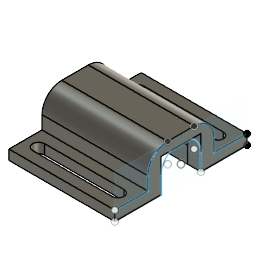
20mmMotorTutucu (Autodesk Fusion 360 design; units mm, degrees)
Autodesk Fusion 360 part; units mm, degrees
sketch "Eskiz1" plane through (0, 0, 0) normal (0, 0, 1) x (1, 0, 0)
  line L0 (0, 5) -> (32, 5) construction
  line L1 (32, 40) -> (0, 40)
  line L2 (32, 0) -> (32, 40)
  line L3 (0, 0) -> (32, 0)
  line L4 (28, 40) -> (28, 0) construction
  line L5 (4, 40) -> (4, 0) construction
  line L6 (0, 35) -> (32, 35) construction
  line L7 (0, 40) -> (0, 0)
  line L8 (4, 6.8) -> (28, 6.8)
  line L9 (28, 3.2) -> (4, 3.2)
  line L10 (4, 36.8) -> (28, 36.8)
  line L11 (28, 33.2) -> (4, 33.2)
  arc A0 (4, 36.8) -> (4, 33.2) centre (4, 35) ccw
  arc A1 (28, 33.2) -> (28, 36.8) centre (28, 35) ccw
  arc A2 (4, 6.8) -> (4, 3.2) centre (4, 5) ccw
  arc A3 (28, 3.2) -> (28, 6.8) centre (28, 5) ccw
  dimension "d4" = 3.6
  dimension "d5" = 3.6
  dimension "d6" = 3.6
  dimension "d7" = 3.6
  constraint horizontal L3
  constraint vertical L2
  constraint horizontal L1
  constraint vertical L7
  constraint coincident L0.start L7
  constraint coincident L0.end L2
  constraint perpendicular L0 L2
  constraint coincident L6.start L7
  constraint coincident L6.end L2
  constraint perpendicular L2 L6
  constraint coincident L5.start L1
  constraint coincident L5.end L3
  constraint perpendicular L3 L5
  constraint coincident L4.start L1
  constraint coincident L4.end L3
  constraint perpendicular L3 L4
  constraint coincident A0.centre L5
  constraint coincident A0.centre L6
  constraint coincident A1.centre L6
  constraint coincident A1.centre L4
  constraint coincident A2.centre L0
  constraint coincident A2.centre L5
  constraint coincident A3.centre L0
  constraint coincident A3.centre L4
  constraint coincident L3.start L7.end
  constraint coincident L5 L8.start
  constraint coincident L4 L8.end
  constraint coincident L4 L9.start
  constraint coincident L5 L9.end
  constraint tangent L9 A2
  constraint coincident L5 L10.start
  constraint coincident L4 L10.end
  constraint tangent L10 A1
  constraint coincident L4 L11.start
  constraint coincident L5 L11.end
  constraint tangent L11 A0
  measures "d4" diameter of A0
  measures "d5" diameter of A1
  measures "d6" diameter of A2
  measures "d7" diameter of A3
extrude "Ekstrüzyon1" add sketch "Eskiz1" along normal blind 13
sketch "Eskiz3" plane through (32, 0, 0) normal (1, 0, 0) x (0, 1, 0)
  line L0 (0, 0) -> (40, 0)
  line L1 (40, 0) -> (40, 13)
  line L2 (40, 13) -> (0, 13)
  line L3 (0, 13) -> (0, 0)
  line L4 (14, 5) -> (14, 0)
  line L5 (26, 5) -> (26, 0)
  line L6 (40, 0) -> (26, 0)
  line L7 (14, 0) -> (0, 0)
  line L8 (10, 7) -> (10, 2.9923)
  line L9 (30, 7) -> (30, 3.1179)
  arc A0 (16, 13) -> (10, 7) centre (16, 7) ccw
  line L10 (0, 3) -> (10, 2.9923)
  line L11 (30, 3.1179) -> (40, 3)
  arc A1 (30, 7) -> (24, 13) centre (24, 7) ccw
  line L12 (26, 0) -> (26, 5)
  line L13 (23.3166, 10) -> (16.6834, 10)
  line L14 (14, 5) -> (14, 0)
  arc A2 (26, 5) -> (23.3166, 10) centre (20, 5) ccw
  arc A3 (16.6834, 10) -> (14, 5) centre (20, 5) ccw
  dimension "d32" = 3
  dimension "d35" = 6
  dimension "d45" = 3
  constraint horizontal L6
  constraint coincident L0.end L1.start
  constraint coincident L4.end L6
  constraint collinear L6 L7
  constraint coincident L1 L11.end
  constraint perpendicular L7 L8
  constraint perpendicular L0 L9
  constraint tangent L8 A0
  constraint tangent L2 A0
  constraint coincident L2 A0.start
  constraint coincident L2 A1.end
  constraint vertical L12
  constraint horizontal L13
  constraint vertical L14
  constraint concentric A2 A3
  measures "d32" distance of L0.start L10.start
  measures "d35" radius of A0
  measures "d45" distance of L0.end L11.end
extrude "Ekstrüzyon4" cut sketch "Eskiz3" against normal blind 40 contours L0 L4 L5 L12 L13 L14 A2 A3 | L2 L3 L8 A0 L10 | L1 L2 L9 L11 A1
sketch "Eskiz4" plane through (32, 0, 0) normal (1, 0, 0) x (0, 1, 0)
  line L0 (14.0094, 0.0419) -> (26.0094, 0.0419)
  line L1 (26.0094, 0.0419) -> (26.0094, 10.0419)
  line L2 (26.0094, 10.0419) -> (14.0094, 10.0419)
  line L3 (14.0094, 10.0419) -> (14.0094, 0.0419)
  line L4 (0, 3) -> (39.9773, 3)
  dimension "d39" = 12
  dimension "d40" = 10
  dimension "d44" = 3
  constraint horizontal L0
  constraint vertical L1
  constraint horizontal L2
  constraint vertical L3
  constraint perpendicular L1 L4
  measures "d39" distance of L0.start L0.end
  measures "d40" distance of L0.start L2.end
  measures "d44" distance of L4.start origin
extrude "Ekstrüzyon5" cut sketch "Eskiz4" against normal blind 4
sketch "Eskiz5" plane through (32, 0, 0) normal (1, 0, 0) x (0, 1, 0)
